Autodesk Fusion 360 part; units mm, degrees
note: some values were not read from the file. Set by a fixed rule: which sketch regions a step uses.
(part 2 of 3)
  line L947 (26.0919, -13.4081) -> (26.0919, -6.5919)
  line L948 (-3.9115, -47.833) -> (-4.0885, -47.833)
  line L949 (-3.9115, -40.0885) -> (-3.9115, -47.833)
  line L950 (-2, -40.0885) -> (-3.9115, -40.0885)
  line L951 (-2, -39.9115) -> (-2, -40.0885)
  line L952 (-3.9115, -39.9115) -> (-2, -39.9115)
  line L953 (-3.9115, -40.0885) -> (-3.9115, -39.9115)
  line L954 (-4.0885, -40.0885) -> (-3.9115, -40.0885)
  line L955 (-4.0885, -39.9115) -> (-4.0885, -40.0885)
  line L956 (-10.9115, -39.9115) -> (-4.0885, -39.9115)
  line L957 (-10.9115, -40.0885) -> (-10.9115, -39.9115)
  line L958 (-11.0885, -40.0885) -> (-10.9115, -40.0885)
  line L959 (-11.0885, -39.9115) -> (-11.0885, -40.0885)
  line L960 (-17.9115, -39.9115) -> (-11.0885, -39.9115)
  line L961 (-17.9115, -40.0885) -> (-17.9115, -39.9115)
  line L962 (-18.0885, -40.0885) -> (-17.9115, -40.0885)
  line L963 (-18.0885, -39.9115) -> (-18.0885, -40.0885)
  line L964 (-17.9115, -39.9115) -> (-18.0885, -39.9115)
  line L965 (-11.0885, -39.9115) -> (-17.9115, -39.9115)
  line L966 (-10.9115, -39.9115) -> (-11.0885, -39.9115)
  line L967 (-4.0885, -39.9115) -> (-10.9115, -39.9115)
  line L968 (-3.9115, -39.9115) -> (-4.0885, -39.9115)
  line L969 (-2, -39.9115) -> (-3.9115, -39.9115)
  line L970 (-3.9115, -39.9115) -> (-2, -39.9115)
  line L971 (-3.9115, -28.0885) -> (-3.9115, -39.9115)
  line L972 (-4.0885, -28.0885) -> (-3.9115, -28.0885)
  line L973 (-4.0885, -39.9115) -> (-4.0885, -28.0885)
  line L974 (-10.9115, -39.9115) -> (-4.0885, -39.9115)
  line L975 (-10.9115, -28.0885) -> (-10.9115, -39.9115)
  line L976 (-11.0885, -28.0885) -> (-10.9115, -28.0885)
  line L977 (-11.0885, -39.9115) -> (-11.0885, -28.0885)
  line L978 (-17.9115, -39.9115) -> (-11.0885, -39.9115)
  line L979 (-17.9115, -28.0885) -> (-17.9115, -39.9115)
  line L980 (-18.0885, -28.0885) -> (-17.9115, -28.0885)
  line L981 (-18.0885, -39.9115) -> (-18.0885, -28.0885)
  line L982 (-24.9115, -39.9115) -> (-18.0885, -39.9115)
  line L983 (-24.9115, -28.0885) -> (-24.9115, -39.9115)
  line L984 (-18.0885, -28.0885) -> (-24.9115, -28.0885)
  line L985 (-17.9115, -28.0885) -> (-18.0885, -28.0885)
  line L986 (-11.0885, -28.0885) -> (-17.9115, -28.0885)
  line L987 (-10.9115, -28.0885) -> (-11.0885, -28.0885)
  line L988 (-4.0885, -28.0885) -> (-10.9115, -28.0885)
  line L989 (-3.9115, -28.0885) -> (-4.0885, -28.0885)
  line L990 (-2, -28.0885) -> (-3.9115, -28.0885)
  line L991 (-2, -27.9115) -> (-2, -28.0885)
  line L992 (-3.9115, -27.9115) -> (-2, -27.9115)
  line L993 (-3.9115, -28.0885) -> (-3.9115, -27.9115)
  line L994 (-4.0885, -28.0885) -> (-3.9115, -28.0885)
  line L995 (-4.0885, -27.9115) -> (-4.0885, -28.0885)
  line L996 (-10.9115, -27.9115) -> (-4.0885, -27.9115)
  line L997 (-10.9115, -28.0885) -> (-10.9115, -27.9115)
  line L998 (-11.0885, -28.0885) -> (-10.9115, -28.0885)
  line L999 (-11.0885, -27.9115) -> (-11.0885, -28.0885)
  line L1000 (-17.9115, -27.9115) -> (-11.0885, -27.9115)
  line L1001 (-17.9115, -28.0885) -> (-17.9115, -27.9115)
  line L1002 (-18.0885, -28.0885) -> (-17.9115, -28.0885)
  line L1003 (-18.0885, -27.9115) -> (-18.0885, -28.0885)
  line L1004 (-24.9115, -27.9115) -> (-18.0885, -27.9115)
  line L1005 (-24.9115, -28.0885) -> (-24.9115, -27.9115)
  line L1006 (-25.0885, -28.0885) -> (-24.9115, -28.0885)
  line L1007 (-25.0885, -27.9115) -> (-25.0885, -28.0885)
  line L1008 (-31.9115, -27.9115) -> (-25.0885, -27.9115)
  line L1009 (-31.9115, -28.0885) -> (-31.9115, -27.9115)
  line L1010 (-32.0885, -28.0885) -> (-31.9115, -28.0885)
  line L1011 (-32.0885, -27.9115) -> (-32.0885, -28.0885)
  line L1012 (-38.9115, -27.9115) -> (-32.0885, -27.9115)
  line L1013 (-38.9115, -27.9821) -> (-38.9115, -27.9115)
  line L1014 (-38.9872, -27.9821) -> (-38.9115, -27.9821)
  line L1015 (-38.9872, -27.9115) -> (-38.9872, -27.9821)
  line L1016 (-38.9115, -27.9115) -> (-38.9872, -27.9115)
  line L1017 (-32.0885, -27.9115) -> (-38.9115, -27.9115)
  line L1018 (-31.9115, -27.9115) -> (-32.0885, -27.9115)
  line L1019 (-25.0885, -27.9115) -> (-31.9115, -27.9115)
  line L1020 (-24.9115, -27.9115) -> (-25.0885, -27.9115)
  line L1021 (-18.0885, -27.9115) -> (-24.9115, -27.9115)
  line L1022 (-17.9115, -27.9115) -> (-18.0885, -27.9115)
  line L1023 (-11.0885, -27.9115) -> (-17.9115, -27.9115)
  line L1024 (-10.9115, -27.9115) -> (-11.0885, -27.9115)
  line L1025 (-4.0885, -27.9115) -> (-10.9115, -27.9115)
  line L1026 (-3.9115, -27.9115) -> (-4.0885, -27.9115)
  line L1027 (-2, -27.9115) -> (-3.9115, -27.9115)
  line L1028 (-3.9115, -27.9115) -> (-2, -27.9115)
  line L1029 (-3.9115, -16.0885) -> (-3.9115, -27.9115)
  line L1030 (-4.0885, -16.0885) -> (-3.9115, -16.0885)
  line L1031 (-4.0885, -27.9115) -> (-4.0885, -16.0885)
  line L1032 (-10.9115, -27.9115) -> (-4.0885, -27.9115)
  line L1033 (-10.9115, -16.0885) -> (-10.9115, -27.9115)
  line L1034 (-11.0885, -16.0885) -> (-10.9115, -16.0885)
  line L1035 (-11.0885, -27.9115) -> (-11.0885, -16.0885)
  line L1036 (-17.9115, -27.9115) -> (-11.0885, -27.9115)
  line L1037 (-17.9115, -16.0885) -> (-17.9115, -27.9115)
  line L1038 (-18.0885, -16.0885) -> (-17.9115, -16.0885)
  line L1039 (-18.0885, -27.9115) -> (-18.0885, -16.0885)
  line L1040 (-24.9115, -27.9115) -> (-18.0885, -27.9115)
  line L1041 (-24.9115, -16.0885) -> (-24.9115, -27.9115)
  line L1042 (-25.0885, -16.0885) -> (-24.9115, -16.0885)
  line L1043 (-25.0885, -27.9115) -> (-25.0885, -16.0885)
  line L1044 (-31.9115, -27.9115) -> (-25.0885, -27.9115)
  line L1045 (-31.9115, -16.0885) -> (-31.9115, -27.9115)
  line L1046 (-32.0885, -16.0885) -> (-31.9115, -16.0885)
  line L1047 (-32.0885, -27.9115) -> (-32.0885, -16.0885)
  line L1048 (-38.9115, -27.9115) -> (-32.0885, -27.9115)
  line L1049 (-38.9115, -16.0885) -> (-38.9115, -27.9115)
  line L1050 (-32.0885, -16.0885) -> (-38.9115, -16.0885)
  line L1051 (-31.9115, -16.0885) -> (-32.0885, -16.0885)
  line L1052 (-25.0885, -16.0885) -> (-31.9115, -16.0885)
  line L1053 (-24.9115, -16.0885) -> (-25.0885, -16.0885)
  line L1054 (-18.0885, -16.0885) -> (-24.9115, -16.0885)
  line L1055 (-17.9115, -16.0885) -> (-18.0885, -16.0885)
  line L1056 (-11.0885, -16.0885) -> (-17.9115, -16.0885)
  line L1057 (-10.9115, -16.0885) -> (-11.0885, -16.0885)
  line L1058 (-4.0885, -16.0885) -> (-10.9115, -16.0885)
  line L1059 (-3.9115, -16.0885) -> (-4.0885, -16.0885)
  line L1060 (-2, -16.0885) -> (-3.9115, -16.0885)
  line L1061 (-2, -15.9115) -> (-2, -16.0885)
  line L1062 (-3.9115, -15.9115) -> (-2, -15.9115)
  line L1063 (-3.9115, -16.0885) -> (-3.9115, -15.9115)
  line L1064 (-4.0885, -16.0885) -> (-3.9115, -16.0885)
  line L1065 (-4.0885, -15.9115) -> (-4.0885, -16.0885)
  line L1066 (-10.9115, -15.9115) -> (-4.0885, -15.9115)
  line L1067 (-10.9115, -16.0885) -> (-10.9115, -15.9115)
  line L1068 (-11.0885, -16.0885) -> (-10.9115, -16.0885)
  line L1069 (-11.0885, -15.9115) -> (-11.0885, -16.0885)
  line L1070 (-17.9115, -15.9115) -> (-11.0885, -15.9115)
  line L1071 (-17.9115, -16.0885) -> (-17.9115, -15.9115)
  line L1072 (-18.0885, -16.0885) -> (-17.9115, -16.0885)
  line L1073 (-18.0885, -15.9115) -> (-18.0885, -16.0885)
  line L1074 (-24.9115, -15.9115) -> (-18.0885, -15.9115)
  line L1075 (-24.9115, -16.0885) -> (-24.9115, -15.9115)
  line L1076 (-25.0885, -16.0885) -> (-24.9115, -16.0885)
  line L1077 (-25.0885, -15.9115) -> (-25.0885, -16.0885)
  line L1078 (-31.9115, -15.9115) -> (-25.0885, -15.9115)
  line L1079 (-31.9115, -16.0885) -> (-31.9115, -15.9115)
  line L1080 (-32.0885, -16.0885) -> (-31.9115, -16.0885)
  line L1081 (-32.0885, -15.9115) -> (-32.0885, -16.0885)
  line L1082 (-31.9115, -15.9115) -> (-32.0885, -15.9115)
  line L1083 (-25.0885, -15.9115) -> (-31.9115, -15.9115)
  line L1084 (-24.9115, -15.9115) -> (-25.0885, -15.9115)
  line L1085 (-18.0885, -15.9115) -> (-24.9115, -15.9115)
  line L1086 (-17.9115, -15.9115) -> (-18.0885, -15.9115)
  line L1087 (-11.0885, -15.9115) -> (-17.9115, -15.9115)
  line L1088 (3.9115, -47.833) -> (3.9115, -40.0885)
  line L1089 (3.9115, -40.0885) -> (2, -40.0885)
  line L1090 (2, -40.0885) -> (2, -39.9115)
  line L1091 (2, -39.9115) -> (3.9115, -39.9115)
  line L1092 (3.9115, -39.9115) -> (3.9115, -40.0885)
  line L1093 (3.9115, -40.0885) -> (4.0885, -40.0885)
  line L1094 (4.0885, -40.0885) -> (4.0885, -39.9115)
  line L1095 (4.0885, -39.9115) -> (10.9115, -39.9115)
  line L1096 (10.9115, -39.9115) -> (10.9115, -40.0885)
  line L1097 (10.9115, -40.0885) -> (11.0885, -40.0885)
  line L1098 (11.0885, -40.0885) -> (11.0885, -39.9115)
  line L1099 (11.0885, -39.9115) -> (17.9115, -39.9115)
  line L1100 (17.9115, -39.9115) -> (17.9115, -40.0885)
  line L1101 (17.9115, -40.0885) -> (18.0885, -40.0885)
  line L1102 (18.0885, -40.0885) -> (18.0885, -39.9115)
  line L1103 (18.0885, -39.9115) -> (17.9115, -39.9115)
  line L1104 (17.9115, -39.9115) -> (11.0885, -39.9115)
  line L1105 (11.0885, -39.9115) -> (10.9115, -39.9115)
  line L1106 (10.9115, -39.9115) -> (4.0885, -39.9115)
  line L1107 (4.0885, -39.9115) -> (3.9115, -39.9115)
  line L1108 (3.9115, -39.9115) -> (2, -39.9115)
  line L1109 (2, -39.9115) -> (3.9115, -39.9115)
  line L1110 (3.9115, -39.9115) -> (3.9115, -28.0885)
  line L1111 (3.9115, -28.0885) -> (4.0885, -28.0885)
  line L1112 (4.0885, -28.0885) -> (4.0885, -39.9115)
  line L1113 (4.0885, -39.9115) -> (10.9115, -39.9115)
  line L1114 (10.9115, -39.9115) -> (10.9115, -28.0885)
  line L1115 (10.9115, -28.0885) -> (11.0885, -28.0885)
  line L1116 (11.0885, -28.0885) -> (11.0885, -39.9115)
  line L1117 (11.0885, -39.9115) -> (17.9115, -39.9115)
  line L1118 (17.9115, -39.9115) -> (17.9115, -28.0885)
  line L1119 (17.9115, -28.0885) -> (18.0885, -28.0885)
  line L1120 (18.0885, -28.0885) -> (18.0885, -39.9115)
  line L1121 (18.0885, -39.9115) -> (24.9115, -39.9115)
  line L1122 (24.9115, -39.9115) -> (24.9115, -28.0885)
  line L1123 (24.9115, -28.0885) -> (18.0885, -28.0885)
  line L1124 (18.0885, -28.0885) -> (17.9115, -28.0885)
  line L1125 (17.9115, -28.0885) -> (11.0885, -28.0885)
  line L1126 (11.0885, -28.0885) -> (10.9115, -28.0885)
  line L1127 (10.9115, -28.0885) -> (4.0885, -28.0885)
  line L1128 (4.0885, -28.0885) -> (3.9115, -28.0885)
  line L1129 (3.9115, -28.0885) -> (2, -28.0885)
  line L1130 (2, -28.0885) -> (2, -27.9115)
  line L1131 (2, -27.9115) -> (3.9115, -27.9115)
  line L1132 (3.9115, -27.9115) -> (3.9115, -28.0885)
  line L1133 (3.9115, -28.0885) -> (4.0885, -28.0885)
  line L1134 (4.0885, -28.0885) -> (4.0885, -27.9115)
  line L1135 (4.0885, -27.9115) -> (10.9115, -27.9115)
  line L1136 (10.9115, -27.9115) -> (10.9115, -28.0885)
  line L1137 (10.9115, -28.0885) -> (11.0885, -28.0885)
  line L1138 (11.0885, -28.0885) -> (11.0885, -27.9115)
  line L1139 (11.0885, -27.9115) -> (17.9115, -27.9115)
  line L1140 (17.9115, -27.9115) -> (17.9115, -28.0885)
  line L1141 (17.9115, -28.0885) -> (18.0885, -28.0885)
  line L1142 (18.0885, -28.0885) -> (18.0885, -27.9115)
  line L1143 (18.0885, -27.9115) -> (24.9115, -27.9115)
  line L1144 (24.9115, -27.9115) -> (24.9115, -28.0885)
  line L1145 (24.9115, -28.0885) -> (25.0885, -28.0885)
  line L1146 (25.0885, -28.0885) -> (25.0885, -27.9115)
  line L1147 (25.0885, -27.9115) -> (31.9115, -27.9115)
  line L1148 (31.9115, -27.9115) -> (31.9115, -28.0885)
  line L1149 (31.9115, -28.0885) -> (32.0885, -28.0885)
  line L1150 (32.0885, -28.0885) -> (32.0885, -27.9115)
  line L1151 (32.0885, -27.9115) -> (38.9115, -27.9115)
  line L1152 (38.9115, -27.9115) -> (38.9115, -27.9821)
  line L1153 (38.9115, -27.9821) -> (38.9872, -27.9821)
  line L1154 (38.9872, -27.9821) -> (38.9872, -27.9115)
  line L1155 (38.9872, -27.9115) -> (38.9115, -27.9115)
  line L1156 (38.9115, -27.9115) -> (32.0885, -27.9115)
  line L1157 (32.0885, -27.9115) -> (31.9115, -27.9115)
  line L1158 (31.9115, -27.9115) -> (25.0885, -27.9115)
  line L1159 (25.0885, -27.9115) -> (24.9115, -27.9115)
  line L1160 (24.9115, -27.9115) -> (18.0885, -27.9115)
  line L1161 (18.0885, -27.9115) -> (17.9115, -27.9115)
  line L1162 (17.9115, -27.9115) -> (11.0885, -27.9115)
  line L1163 (11.0885, -27.9115) -> (10.9115, -27.9115)
  line L1164 (10.9115, -27.9115) -> (4.0885, -27.9115)
  line L1165 (4.0885, -27.9115) -> (3.9115, -27.9115)
  line L1166 (3.9115, -27.9115) -> (2, -27.9115)
  line L1167 (2, -27.9115) -> (3.9115, -27.9115)
  line L1168 (3.9115, -27.9115) -> (3.9115, -16.0885)
  line L1169 (3.9115, -16.0885) -> (4.0885, -16.0885)
  line L1170 (4.0885, -16.0885) -> (4.0885, -27.9115)
  line L1171 (4.0885, -27.9115) -> (10.9115, -27.9115)
  line L1172 (10.9115, -27.9115) -> (10.9115, -16.0885)
  line L1173 (10.9115, -16.0885) -> (11.0885, -16.0885)
  line L1174 (11.0885, -16.0885) -> (11.0885, -27.9115)
  line L1175 (11.0885, -27.9115) -> (17.9115, -27.9115)
  line L1176 (17.9115, -27.9115) -> (17.9115, -16.0885)
  line L1177 (17.9115, -16.0885) -> (18.0885, -16.0885)
  line L1178 (18.0885, -16.0885) -> (18.0885, -27.9115)
  line L1179 (18.0885, -27.9115) -> (24.9115, -27.9115)
  line L1180 (24.9115, -27.9115) -> (24.9115, -16.0885)
  line L1181 (24.9115, -16.0885) -> (25.0885, -16.0885)
  line L1182 (25.0885, -16.0885) -> (25.0885, -27.9115)
  line L1183 (25.0885, -27.9115) -> (31.9115, -27.9115)
  line L1184 (31.9115, -27.9115) -> (31.9115, -16.0885)
  line L1185 (31.9115, -16.0885) -> (32.0885, -16.0885)
  line L1186 (32.0885, -16.0885) -> (32.0885, -27.9115)
  line L1187 (32.0885, -27.9115) -> (38.9115, -27.9115)
  line L1188 (38.9115, -27.9115) -> (38.9115, -16.0885)
  line L1189 (38.9115, -16.0885) -> (32.0885, -16.0885)
  line L1190 (32.0885, -16.0885) -> (31.9115, -16.0885)
  line L1191 (31.9115, -16.0885) -> (25.0885, -16.0885)
  line L1192 (25.0885, -16.0885) -> (24.9115, -16.0885)
  line L1193 (24.9115, -16.0885) -> (18.0885, -16.0885)
  line L1194 (18.0885, -16.0885) -> (17.9115, -16.0885)
  line L1195 (17.9115, -16.0885) -> (11.0885, -16.0885)
  line L1196 (11.0885, -16.0885) -> (10.9115, -16.0885)
  line L1197 (10.9115, -16.0885) -> (4.0885, -16.0885)
  line L1198 (4.0885, -16.0885) -> (3.9115, -16.0885)
  line L1199 (3.9115, -16.0885) -> (2, -16.0885)
  line L1200 (2, -16.0885) -> (2, -15.9115)
  line L1201 (2, -15.9115) -> (3.9115, -15.9115)
  line L1202 (3.9115, -15.9115) -> (3.9115, -16.0885)
  line L1203 (3.9115, -16.0885) -> (4.0885, -16.0885)
  line L1204 (4.0885, -16.0885) -> (4.0885, -15.9115)
  line L1205 (4.0885, -15.9115) -> (10.9115, -15.9115)
  line L1206 (10.9115, -15.9115) -> (10.9115, -16.0885)
  line L1207 (10.9115, -16.0885) -> (11.0885, -16.0885)
  line L1208 (11.0885, -16.0885) -> (11.0885, -15.9115)
  line L1209 (11.0885, -15.9115) -> (17.9115, -15.9115)
  line L1210 (17.9115, -15.9115) -> (17.9115, -16.0885)
  line L1211 (17.9115, -16.0885) -> (18.0885, -16.0885)
  line L1212 (18.0885, -16.0885) -> (18.0885, -15.9115)
  line L1213 (18.0885, -15.9115) -> (24.9115, -15.9115)
  line L1214 (24.9115, -15.9115) -> (24.9115, -16.0885)
  line L1215 (24.9115, -16.0885) -> (25.0885, -16.0885)
  line L1216 (25.0885, -16.0885) -> (25.0885, -15.9115)
  line L1217 (-24.9115, -3.9115) -> (-25.0885, -3.9115)
  line L1218 (-32.0885, -2) -> (-31.9115, -2)
  line L1219 (-17.9115, -3.9115) -> (-11.0885, -3.9115)
  line L1220 (-4.0885, -4.0885) -> (-3.9115, -4.0885)
  line L1221 (-2, -4.0885) -> (-3.9115, -4.0885)
  line L1222 (-3.9115, -3.9115) -> (-4.0885, -3.9115)
  line L1223 (-11.0885, -4.0885) -> (-17.9115, -4.0885)
  line L1224 (-25.0885, -4.0885) -> (-31.9115, -4.0885)
  line L1225 (-18.0885, -40.0885) -> (-24.9115, -40.0885)
  line L1226 (-18.0885, -3.9115) -> (-18.0885, -4.0885)
  line L1227 (-38.9872, -28.0885) -> (-38.9872, -27.9821)
  line L1228 (-31.9115, -3.9115) -> (-32.0885, -3.9115)
  line L1229 (-38.9115, -3.9115) -> (-39.0885, -3.9115)
  line L1230 (-45.9115, -3.9115) -> (-39.0885, -3.9115)
  line L1231 (-38.9115, -15.9115) -> (-39.0885, -15.9115)
  line L1232 (-45.9115, -4.0885) -> (-45.9115, -3.9115)
  line L1233 (-3.9115, -3.9115) -> (-2, -3.9115)
  line L1234 (-18.0885, -3.9115) -> (-24.9115, -3.9115)
  line L1235 (-38.9115, -15.9115) -> (-32.0885, -15.9115)
  line L1236 (-31.9115, -35.7771) -> (-32.0885, -35.7771)
  line L1237 (-32.0885, -28.0885) -> (-38.9872, -28.0885)
  line L1238 (-31.9115, -28.0885) -> (-31.9115, -35.7771)
  line L1239 (-18.0885, -15.9115) -> (-18.0885, -4.0885)
  line L1240 (-3.9115, -2) -> (-3.9115, -3.9115)
  line L1241 (-11.0885, -3.9115) -> (-11.0885, -2)
  line L1242 (-24.9115, -4.0885) -> (-25.0885, -4.0885)
  line L1243 (-4.0885, -4.0885) -> (-10.9115, -4.0885)
  line L1244 (-18.0885, -4.0885) -> (-17.9115, -4.0885)
  line L1245 (-11.0885, -4.0885) -> (-10.9115, -4.0885)
  line L1246 (-31.9115, -3.9115) -> (-25.0885, -3.9115)
  line L1247 (-10.9115, -3.9115) -> (-11.0885, -3.9115)
  line L1248 (-25.0885, -3.9115) -> (-25.0885, -2)
  line L1249 (-2, -3.9115) -> (-2, -4.0885)
  line L1250 (-17.9115, -40.0885) -> (-17.9115, -44.4972)
  line L1251 (-18.0885, -4.0885) -> (-17.9115, -4.0885)
  line L1252 (-47.833, -4.0885) -> (-47.833, -3.9115)
  line L1253 (-3.9115, -4.0885) -> (-4.0885, -4.0885)
  line L1254 (-38.9115, -3.9115) -> (-32.0885, -3.9115)
  line L1255 (-31.9115, -4.0885) -> (-31.9115, -3.9115)
  line L1256 (-39.0885, -16.0885) -> (-45.2548, -16.0885)
  line L1257 (-3.9115, -3.9115) -> (-2, -3.9115)
  line L1258 (-3.9115, -15.9115) -> (-2, -15.9115)
  line L1259 (-32.0885, -3.9115) -> (-38.9115, -3.9115)
  line L1260 (-4.0885, -3.9115) -> (-10.9115, -3.9115)
  line L1261 (-31.9115, -3.9115) -> (-25.0885, -3.9115)
  line L1262 (-32.0885, -3.9115) -> (-32.0885, -2)
  line L1263 (-3.9115, -4.0885) -> (-3.9115, -3.9115)
  line L1264 (-24.9115, -2) -> (-24.9115, -3.9115)
  line L1265 (-31.9115, -15.9115) -> (-25.0885, -15.9115)
  line L1266 (-17.9115, -2) -> (-17.9115, -3.9115)
  line L1267 (-39.0885, -27.9821) -> (-39.0885, -16.0885)
  line L1268 (-26.533, -40.0885) -> (-26.533, -39.9115)
  line L1269 (-46.0885, -3.9115) -> (-46.0885, -4.0885)
  line L1270 (-47.833, -3.9115) -> (-46.0885, -3.9115)
  line L1271 (-17.9115, -3.9115) -> (-18.0885, -3.9115)
  line L1272 (-45.9115, -4.0885) -> (-45.9115, -13.7113)
  line L1273 (-10.9115, -3.9115) -> (-4.0885, -3.9115)
  line L1274 (-25.0885, -40.9756) -> (-25.0885, -40.0885)
  line L1275 (-39.0885, -3.9115) -> (-39.0885, -4.0885)
  line L1276 (-17.9115, -4.0885) -> (-18.0885, -4.0885)
  line L1277 (-11.0885, -15.9115) -> (-11.0885, -4.0885)
  line L1278 (-38.9115, -16.0885) -> (-38.9115, -15.9115)
  line L1279 (-18.0885, -2) -> (-17.9115, -2)
  line L1280 (-4.0885, -4.0885) -> (-3.9115, -4.0885)
  line L1281 (-38.9115, -4.0885) -> (-38.9115, -3.9115)
  line L1282 (-32.0885, -4.0885) -> (-38.9115, -4.0885)
  line L1283 (-46.0885, -4.0885) -> (-45.9115, -4.0885)
  line L1284 (-25.0885, -3.9115) -> (-31.9115, -3.9115)
  line L1285 (-24.9115, -3.9115) -> (-18.0885, -3.9115)
  line L1286 (-24.9115, -39.9115) -> (-25.0885, -39.9115)
  line L1287 (-26.533, -39.9115) -> (-25.0885, -39.9115)
  line L1288 (-39.0885, -15.9115) -> (-39.0885, -16.0885)
  line L1289 (-24.9115, -4.0885) -> (-24.9115, -3.9115)
  line L1290 (-25.0885, -39.9115) -> (-25.0885, -40.0885)
  line L1291 (-10.9115, -4.0885) -> (-10.9115, -3.9115)
  line L1292 (-31.9115, -4.0885) -> (-32.0885, -4.0885)
  line L1293 (-25.0885, -40.0885) -> (-24.9115, -40.0885)
  line L1294 (-25.0885, -4.0885) -> (-24.9115, -4.0885)
  line L1295 (-38.9872, -27.9821) -> (-39.0885, -27.9821)
  line L1296 (-45.2548, -16.0885) -> (-45.2548, -15.9115)
  line L1297 (-11.0885, -3.9115) -> (-17.9115, -3.9115)
  line L1298 (-32.0885, -15.9115) -> (-32.0885, -4.0885)
  line L1299 (-25.0885, -40.0885) -> (-26.533, -40.0885)
  line L1300 (-45.9115, -2) -> (-45.9115, -3.9115)
  line L1301 (-45.2548, -15.9115) -> (-39.0885, -15.9115)
  line L1302 (-11.0885, -2) -> (-10.9115, -2)
  line L1303 (-46.0885, -13.7113) -> (-46.0885, -4.0885)
  line L1304 (-38.9115, -3.9115) -> (-32.0885, -3.9115)
  line L1305 (-24.9115, -4.0885) -> (-24.9115, -15.9115)
  line L1306 (-25.0885, -4.0885) -> (-24.9115, -4.0885)
  line L1307 (-17.9115, -3.9115) -> (-11.0885, -3.9115)
  line L1308 (-18.0885, -44.4972) -> (-18.0885, -40.0885)
  line L1309 (-10.9115, -4.0885) -> (-10.9115, -15.9115)
  line L1310 (-24.9115, -40.0885) -> (-24.9115, -39.9115)
  line L1311 (-32.0885, -35.7771) -> (-32.0885, -28.0885)
  line L1312 (-18.0885, -4.0885) -> (-24.9115, -4.0885)
  line L1313 (-25.0885, -28.0885) -> (-31.9115, -28.0885)
  line L1314 (-17.9115, -4.0885) -> (-17.9115, -15.9115)
  line L1315 (-17.9115, -44.4972) -> (-18.0885, -44.4972)
  line L1316 (-31.9115, -2) -> (-31.9115, -3.9115)
  line L1317 (-46.0885, -4.0885) -> (-47.833, -4.0885)
  line L1318 (-24.9115, -3.9115) -> (-18.0885, -3.9115)
  line L1319 (-39.0885, -4.0885) -> (-38.9115, -4.0885)
  line L1320 (-25.0885, -2) -> (-24.9115, -2)
  line L1321 (-18.0885, -3.9115) -> (-18.0885, -2)
  line L1322 (-45.9115, -13.7113) -> (-46.0885, -13.7113)
  line L1323 (-2, -3.9115) -> (-3.9115, -3.9115)
  line L1324 (-24.9115, -15.9115) -> (-18.0885, -15.9115)
  line L1325 (-32.0885, -4.0885) -> (-31.9115, -4.0885)
  line L1326 (-38.9115, -4.0885) -> (-38.9115, -15.9115)
  line L1327 (-11.0885, -4.0885) -> (-10.9115, -4.0885)
  line L1328 (-25.0885, -39.9115) -> (-25.0885, -28.0885)
  line L1329 (-24.9115, -40.0885) -> (-24.9115, -40.9756)
  line L1330 (-45.9115, -3.9115) -> (-46.0885, -3.9115)
  line L1331 (-39.0885, -3.9115) -> (-39.0885, -2)
  line L1332 (-10.9115, -15.9115) -> (-4.0885, -15.9115)
  line L1333 (-4.0885, -2) -> (-3.9115, -2)
  line L1334 (-39.0885, -4.0885) -> (-45.9115, -4.0885)
  line L1335 (-46.0885, -2) -> (-45.9115, -2)
  line L1336 (-17.9115, -4.0885) -> (-17.9115, -3.9115)
  line L1337 (-46.0885, -3.9115) -> (-46.0885, -2)
  line L1338 (-38.9115, -2) -> (-38.9115, -3.9115)
  line L1339 (-25.0885, -15.9115) -> (-25.0885, -4.0885)
  line L1340 (-10.9115, -2) -> (-10.9115, -3.9115)
  line L1341 (-32.0885, -3.9115) -> (-32.0885, -4.0885)
  line L1342 (-31.9115, -4.0885) -> (-31.9115, -15.9115)
  line L1343 (-17.9115, -15.9115) -> (-11.0885, -15.9115)
  line L1344 (-39.0885, -2) -> (-38.9115, -2)
  line L1345 (-32.0885, -4.0885) -> (-31.9115, -4.0885)
  line L1346 (-10.9115, -4.0885) -> (-11.0885, -4.0885)
  line L1347 (-24.9115, -40.9756) -> (-25.0885, -40.9756)
  line L1348 (-4.0885, -15.9115) -> (-4.0885, -4.0885)
  line L1349 (-10.9115, -3.9115) -> (-4.0885, -3.9115)
  line L1350 (-11.0885, -3.9115) -> (-11.0885, -4.0885)
  line L1351 (-4.0885, -3.9115) -> (-4.0885, -2)
  line L1352 (-25.0885, -3.9115) -> (-25.0885, -4.0885)
  line L1353 (-39.0885, -15.9115) -> (-39.0885, -4.0885)
  line L1354 (-39.0885, -16.0885) -> (-38.9115, -16.0885)
  line L1355 (-3.9115, -4.0885) -> (-3.9115, -15.9115)
  line L1356 (-4.0885, -3.9115) -> (-4.0885, -4.0885)
  line L1357 (-3.9115, -15.9115) -> (-4.0885, -15.9115)
  line L1358 (-4.0885, -15.9115) -> (-10.9115, -15.9115)
  line L1359 (-2, -15.9115) -> (-3.9115, -15.9115)
  line L1360 (21.1309, 45.3154) -> (23.0874, 44.3505)
  line L1361 (-33.5, -7) -> (-33.5, -13)
  line L1362 (-48.8148, 10.822) -> (-48.2963, 12.941)
  line L1363 (-33.5, -13) -> (-37.5, -13)
  line L1364 (-26.5, 19) -> (-30.5, 19)
  line L1365 (30.5, 19) -> (26.5, 19)
  line L1366 (-5.5, 13) -> (-5.5, 7)
  line L1367 (-30.5, 19) -> (-30.5, 25)
  line L1368 (-9.5, 13) -> (-5.5, 13)
  line L1369 (-30.5, 25) -> (-26.5, 25)
  line L1370 (30.5, 25) -> (30.5, 19)
  line L1371 (-9.5, 7) -> (-9.5, 13)
  line L1372 (37.5, 7) -> (33.5, 7)
  line L1373 (-37.5, -7) -> (-33.5, -7)
  line L1374 (33.5, 13) -> (37.5, 13)
  line L1375 (-5.5, -19) -> (-5.5, -25)
  line L1376 (37.5, 13) -> (37.5, 7)
  line L1377 (-37.5, -13) -> (-37.5, -7)
  line L1378 (-5.5, 7) -> (-9.5, 7)
  line L1379 (-5.5, -25) -> (-9.5, -25)
  line L1380 (-48.2963, 12.941) -> (-47.6858, 15.0353)
  line L1381 (26.5, 25) -> (30.5, 25)
  line L1382 (26.5, 19) -> (26.5, 25)
  line L1383 (-26.5, 25) -> (-26.5, 19)
  line L1384 (-9.5, -19) -> (-5.5, -19)
  line L1385 (-9.5, -25) -> (-9.5, -19)
  line L1386 (23.5, -37) -> (19.5, -37)
  line L1387 (-48.2963, -12.941) -> (-48.8148, -10.822)
  line L1388 (-42.1696, -26.865) -> (-43.3013, -25)
  line L1389 (-46.194, -19.1342) -> (-46.9846, -17.101)
  line L1390 (-46.9846, -17.101) -> (-47.6858, -15.0353)
  line L1391 (-45.3154, -21.1309) -> (-46.194, -19.1342)
  line L1392 (-44.3505, -23.0874) -> (-45.3154, -21.1309)
  line L1393 (-43.3013, -25) -> (-44.3505, -23.0874)
  line L1394 (-47.6858, -15.0353) -> (-48.2963, -12.941)
  line L1395 (-39.6677, -30.4381) -> (-40.9576, -28.6788)
  line L1396 (-40.9576, -28.6788) -> (-42.1696, -26.865)
  line L1397 (-38.3022, -32.1394) -> (-39.6677, -30.4381)
  line L1398 (43.3013, -25) -> (42.1696, -26.865)
  line L1399 (-49.5722, -6.5263) -> (-49.8097, -4.3578)
  line L1400 (40.9576, -28.6788) -> (39.6677, -30.4381)
  line L1401 (39.6677, -30.4381) -> (38.3022, -32.1394)
  line L1402 (32.1394, -38.3022) -> (30.4381, -39.6677)
  line L1403 (49.8097, -4.3578) -> (49.5722, -6.5263)
  line L1404 (48.8148, -10.822) -> (48.2963, -12.941)
  line L1405 (38.3022, -32.1394) -> (36.8639, -33.7795)
  line L1406 (0, 0) -> (0, -50)
  line L1407 (-48.8148, -10.822) -> (-49.2404, -8.6824)
  line L1408 (33.7795, -36.8639) -> (32.1394, -38.3022)
  line L1409 (36.8639, -33.7795) -> (35.3553, -35.3553)
  line L1410 (35.3553, -35.3553) -> (33.7795, -36.8639)
  line L1411 (49.9524, -2.181) -> (49.8097, -4.3578)
  line L1412 (0, -50) -> (0, 0)
  line L1413 (46.9846, -17.101) -> (46.194, -19.1342)
  line L1414 (42.1696, -26.865) -> (40.9576, -28.6788)
  line L1415 (46.194, -19.1342) -> (45.3154, -21.1309)
  line L1416 (-49.9524, -2.181) -> (-50, 0)
  line L1417 (45.3154, -21.1309) -> (44.3505, -23.0874)
  line L1418 (44.3505, -23.0874) -> (43.3013, -25)
  line L1419 (-49.8097, -4.3578) -> (-49.9524, -2.181)
  line L1420 (0, 0) -> (50, 0)
  line L1421 (50, 0) -> (49.9524, -2.181)
  line L1422 (48.2963, -12.941) -> (47.6858, -15.0353)
  line L1423 (49.2404, -8.6824) -> (48.8148, -10.822)
  line L1424 (-49.2404, -8.6824) -> (-49.5722, -6.5263)
  line L1425 (47.6858, -15.0353) -> (46.9846, -17.101)
  line L1426 (-50, 0) -> (0, 0)
  line L1427 (49.5722, -6.5263) -> (49.2404, -8.6824)
  line L1428 (23.0874, -44.3505) -> (21.1309, -45.3154)
  line L1429 (26.865, -42.1696) -> (25, -43.3013)
  line L1430 (30.4381, -39.6677) -> (28.6788, -40.9576)
  line L1431 (28.6788, -40.9576) -> (26.865, -42.1696)
  line L1432 (25, -43.3013) -> (23.0874, -44.3505)
  line L1433 (21.1309, -45.3154) -> (19.1342, -46.194)
  line L1434 (17.101, -46.9846) -> (15.0353, -47.6858)
  line L1435 (15.0353, -47.6858) -> (12.941, -48.2963)
  line L1436 (10.822, -48.8148) -> (8.6824, -49.2404)
  line L1437 (12.941, -48.2963) -> (10.822, -48.8148)
  line L1438 (8.6824, -49.2404) -> (6.5263, -49.5722)
  line L1439 (19.1342, -46.194) -> (17.101, -46.9846)
  line L1440 (36.8639, -33.7795) -> (35.3553, -35.3553)
  line L1441 (5.5, -13) -> (5.5, -7)
  line L1442 (26.865, -42.1696) -> (25, -43.3013)
  line L1443 (40.9576, -28.6788) -> (39.6677, -30.4381)
  line L1444 (8.6824, -49.2404) -> (6.5263, -49.5722)
  line L1445 (17.101, -46.9846) -> (15.0353, -47.6858)
  line L1446 (38.3022, -32.1394) -> (36.8639, -33.7795)
  line L1447 (23.0874, -44.3505) -> (21.1309, -45.3154)
  line L1448 (15.0353, -47.6858) -> (12.941, -48.2963)
  line L1449 (30.4381, -39.6677) -> (28.6788, -40.9576)
  line L1450 (43.3013, -25) -> (42.1696, -26.865)
  line L1451 (2.181, -49.9524) -> (0, -50)
  line L1452 (28.6788, -40.9576) -> (26.865, -42.1696)
  line L1453 (19.1342, -46.194) -> (17.101, -46.9846)
  line L1454 (19.5, -31) -> (23.5, -31)
  line L1455 (5.5, -7) -> (9.5, -7)
  line L1456 (35.3553, -35.3553) -> (33.7795, -36.8639)
  line L1457 (19.5, -37) -> (19.5, -31)
  line L1458 (44.3505, -23.0874) -> (43.3013, -25)
  line L1459 (6.5263, -49.5722) -> (4.3578, -49.8097)
  line L1460 (33.7795, -36.8639) -> (32.1394, -38.3022)
  line L1461 (4.3578, -49.8097) -> (2.181, -49.9524)
  line L1462 (9.5, -7) -> (9.5, -13)
  line L1463 (32.1394, -38.3022) -> (30.4381, -39.6677)
  line L1464 (21.1309, -45.3154) -> (19.1342, -46.194)
  line L1465 (45.3154, -21.1309) -> (44.3505, -23.0874)
  line L1466 (9.5, -13) -> (5.5, -13)
  line L1467 (39.6677, -30.4381) -> (38.3022, -32.1394)
  line L1468 (12.941, -48.2963) -> (10.822, -48.8148)
  line L1469 (10.822, -48.8148) -> (8.6824, -49.2404)
  line L1470 (25, -43.3013) -> (23.0874, -44.3505)
  line L1471 (23.5, -31) -> (23.5, -37)
  line L1472 (42.1696, -26.865) -> (40.9576, -28.6788)
  line L1473 (49.2404, -8.6824) -> (48.8148, -10.822)
  line L1474 (46.9846, 17.101) -> (47.6858, 15.0353)
  line L1475 (48.2963, 12.941) -> (48.8148, 10.822)
  line L1476 (35.3553, 35.3553) -> (36.8639, 33.7795)
  line L1477 (42.1696, 26.865) -> (43.3013, 25)
  line L1478 (45.3154, 21.1309) -> (46.194, 19.1342)
  line L1479 (49.8097, -4.3578) -> (49.5722, -6.5263)
  line L1480 (39.6677, 30.4381) -> (40.9576, 28.6788)
  line L1481 (48.8148, 10.822) -> (49.2404, 8.6824)
  line L1482 (49.5722, 6.5263) -> (49.8097, 4.3578)
  line L1483 (49.9524, 2.181) -> (50, 0)
  line L1484 (46.194, -19.1342) -> (45.3154, -21.1309)
  line L1485 (47.6858, -15.0353) -> (46.9846, -17.101)
  line L1486 (49.8097, 4.3578) -> (49.9524, 2.181)
  line L1487 (49.5722, -6.5263) -> (49.2404, -8.6824)
  line L1488 (38.3022, 32.1394) -> (39.6677, 30.4381)
  line L1489 (48.2963, -12.941) -> (47.6858, -15.0353)
  line L1490 (46.9846, -17.101) -> (46.194, -19.1342)
  line L1491 (36.8639, 33.7795) -> (38.3022, 32.1394)
  line L1492 (47.6858, 15.0353) -> (48.2963, 12.941)
  line L1493 (33.7795, 36.8639) -> (35.3553, 35.3553)
  line L1494 (43.3013, 25) -> (44.3505, 23.0874)
  line L1495 (50, 0) -> (49.9524, -2.181)
  line L1496 (48.8148, -10.822) -> (48.2963, -12.941)
  line L1497 (40.9576, 28.6788) -> (42.1696, 26.865)
  line L1498 (46.194, 19.1342) -> (46.9846, 17.101)
  line L1499 (49.9524, -2.181) -> (49.8097, -4.3578)
  line L1500 (44.3505, 23.0874) -> (45.3154, 21.1309)
  line L1501 (49.2404, 8.6824) -> (49.5722, 6.5263)
  line L1502 (32.1394, 38.3022) -> (33.7795, 36.8639)
  line L1503 (48.8148, 10.822) -> (49.2404, 8.6824)
  line L1504 (-4.3578, -49.8097) -> (-6.5263, -49.5722)
  line L1505 (-43.3013, 25) -> (-42.1696, 26.865)
  line L1506 (-17.101, 46.9846) -> (-15.0353, 47.6858)
  line L1507 (-49.9524, 2.181) -> (-49.8097, 4.3578)
  line L1508 (-4.3578, 49.8097) -> (-2.181, 49.9524)
  line L1509 (46.9846, 17.101) -> (47.6858, 15.0353)
  line L1510 (-2.181, 49.9524) -> (0, 50)
  line L1511 (8.6824, 49.2404) -> (10.822, 48.8148)
  line L1512 (-49.2404, 8.6824) -> (-48.8148, 10.822)
  line L1513 (-10.822, 48.8148) -> (-8.6824, 49.2404)
  line L1514 (-44.3505, 23.0874) -> (-43.3013, 25)
  line L1515 (-8.6824, 49.2404) -> (-6.5263, 49.5722)
  line L1516 (47.6858, 15.0353) -> (48.2963, 12.941)
  line L1517 (46.194, 19.1342) -> (46.9846, 17.101)
  line L1518 (-49.8097, -4.3578) -> (-49.9524, -2.181)
  line L1519 (-49.5722, 6.5263) -> (-49.2404, 8.6824)
  line L1520 (43.3013, 25) -> (44.3505, 23.0874)
  line L1521 (-25, 43.3013) -> (-23.0874, 44.3505)
  line L1522 (-46.9846, 17.101) -> (-46.194, 19.1342)
  line L1523 (-50, 0) -> (-49.9524, 2.181)
  line L1524 (33.5, 7) -> (33.5, 13)
  line L1525 (-30.4381, 39.6677) -> (-28.6788, 40.9576)
  line L1526 (-49.8097, 4.3578) -> (-49.5722, 6.5263)
  line L1527 (-6.5263, 49.5722) -> (-4.3578, 49.8097)
  line L1528 (-26.865, 42.1696) -> (-25, 43.3013)
  line L1529 (-42.1696, 26.865) -> (-40.9576, 28.6788)
  line L1530 (-39.6677, 30.4381) -> (-38.3022, 32.1394)
  line L1531 (0, -50) -> (-2.181, -49.9524)
  line L1532 (44.3505, 23.0874) -> (45.3154, 21.1309)
  line L1533 (-33.7795, 36.8639) -> (-32.1394, 38.3022)
  line L1534 (19.1342, 46.194) -> (21.1309, 45.3154)
  line L1535 (-46.9846, -17.101) -> (-47.6858, -15.0353)
  line L1536 (-12.941, 48.2963) -> (-10.822, 48.8148)
  line L1537 (-35.3553, 35.3553) -> (-33.7795, 36.8639)
  line L1538 (-19.1342, 46.194) -> (-17.101, 46.9846)
  line L1539 (17.101, 46.9846) -> (19.1342, 46.194)
  line L1540 (6.5263, 49.5722) -> (8.6824, 49.2404)
  line L1541 (-49.8097, 4.3578) -> (-49.5722, 6.5263)
  line L1542 (40.9576, 28.6788) -> (42.1696, 26.865)
  line L1543 (-38.3022, 32.1394) -> (-36.8639, 33.7795)
  line L1544 (48.2963, 12.941) -> (48.8148, 10.822)
  line L1545 (-23.0874, 44.3505) -> (-21.1309, 45.3154)
  line L1546 (42.1696, 26.865) -> (43.3013, 25)
  line L1547 (-49.5722, 6.5263) -> (-49.2404, 8.6824)
  line L1548 (49.2404, 8.6824) -> (49.5722, 6.5263)
  line L1549 (-48.8148, -10.822) -> (-49.2404, -8.6824)
  line L1550 (15.0353, 47.6858) -> (17.101, 46.9846)
  line L1551 (-21.1309, 45.3154) -> (-19.1342, 46.194)
  line L1552 (-28.6788, 40.9576) -> (-26.865, 42.1696)
  line L1553 (45.3154, 21.1309) -> (46.194, 19.1342)
  line L1554 (49.5722, 6.5263) -> (49.8097, 4.3578)
  line L1555 (-2.181, -49.9524) -> (-4.3578, -49.8097)
  line L1556 (-49.9524, -2.181) -> (-50, 0)
  line L1557 (-40.9576, 28.6788) -> (-39.6677, 30.4381)
  line L1558 (39.6677, 30.4381) -> (40.9576, 28.6788)
  line L1559 (-47.6858, -15.0353) -> (-48.2963, -12.941)
  line L1560 (-48.2963, 12.941) -> (-47.6858, 15.0353)
  line L1561 (-49.2404, 8.6824) -> (-48.8148, 10.822)
  line L1562 (-44.3505, -23.0874) -> (-45.3154, -21.1309)
  line L1563 (-50, 0) -> (-49.9524, 2.181)
  line L1564 (-43.3013, -25) -> (-44.3505, -23.0874)
  line L1565 (-30.4381, -39.6677) -> (-32.1394, -38.3022)
  line L1566 (49.8097, 4.3578) -> (49.9524, 2.181)
  line L1567 (-15.0353, -47.6858) -> (-17.101, -46.9846)
  line L1568 (10.822, 48.8148) -> (12.941, 48.2963)
  line L1569 (-36.8639, -33.7795) -> (-38.3022, -32.1394)
  line L1570 (-49.5722, -6.5263) -> (-49.8097, -4.3578)
  line L1571 (-21.1309, -45.3154) -> (-23.0874, -44.3505)
  line L1572 (50, 0) -> (0, 0)
  line L1573 (-49.9524, 2.181) -> (-49.8097, 4.3578)
  line L1574 (-36.8639, 33.7795) -> (-35.3553, 35.3553)
  line L1575 (0, 0) -> (-50, 0)
  line L1576 (-6.5263, -49.5722) -> (-8.6824, -49.2404)
  line L1577 (-12.941, -48.2963) -> (-15.0353, -47.6858)
  line L1578 (-48.2963, -12.941) -> (-48.8148, -10.822)
  line L1579 (-49.2404, -8.6824) -> (-49.5722, -6.5263)
  line L1580 (28.6788, 40.9576) -> (30.4381, 39.6677)
  line L1581 (-32.1394, -38.3022) -> (-33.7795, -36.8639)
  line L1582 (-38.3022, -32.1394) -> (-39.6677, -30.4381)
  line L1583 (-10.822, -48.8148) -> (-12.941, -48.2963)
  line L1584 (26.865, 42.1696) -> (28.6788, 40.9576)
  line L1585 (-40.9576, -28.6788) -> (-42.1696, -26.865)
  line L1586 (-46.194, -19.1342) -> (-46.9846, -17.101)
  line L1587 (-35.3553, -35.3553) -> (-36.8639, -33.7795)
  line L1588 (-39.6677, -30.4381) -> (-40.9576, -28.6788)
  line L1589 (-42.1696, -26.865) -> (-43.3013, -25)
  line L1590 (-45.3154, -21.1309) -> (-46.194, -19.1342)
  line L1591 (36.8639, 33.7795) -> (38.3022, 32.1394)
  line L1592 (-47.6858, 15.0353) -> (-46.9846, 17.101)
  line L1593 (49.9524, 2.181) -> (50, 0)
  line L1594 (-8.6824, -49.2404) -> (-10.822, -48.8148)
  line L1595 (-45.3154, 21.1309) -> (-44.3505, 23.0874)
  line L1596 (12.941, 48.2963) -> (15.0353, 47.6858)
  line L1597 (0, 50) -> (0, 0)
  line L1598 (-32.1394, 38.3022) -> (-30.4381, 39.6677)
  line L1599 (-15.0353, 47.6858) -> (-12.941, 48.2963)
  line L1600 (38.3022, 32.1394) -> (39.6677, 30.4381)
  line L1601 (-48.8148, 10.822) -> (-48.2963, 12.941)
  line L1602 (-46.194, 19.1342) -> (-45.3154, 21.1309)
  line L1603 (35.3553, 35.3553) -> (36.8639, 33.7795)
  line L1604 (23.0874, 44.3505) -> (25, 43.3013)
  line L1605 (-33.7795, -36.8639) -> (-35.3553, -35.3553)
  line L1606 (33.7795, 36.8639) -> (35.3553, 35.3553)
  line L1607 (-17.101, -46.9846) -> (-19.1342, -46.194)
  line L1608 (-19.1342, -46.194) -> (-21.1309, -45.3154)
  line L1609 (25, 43.3013) -> (26.865, 42.1696)
  line L1610 (-26.865, -42.1696) -> (-28.6788, -40.9576)
  line L1611 (-23.0874, -44.3505) -> (-25, -43.3013)
  line L1612 (-28.6788, -40.9576) -> (-30.4381, -39.6677)
  line L1613 (30.4381, 39.6677) -> (32.1394, 38.3022)
  line L1614 (32.1394, 38.3022) -> (33.7795, 36.8639)
  line L1615 (-25, -43.3013) -> (-26.865, -42.1696)
  line L1616 (4.3578, -49.8097) -> (2.181, -49.9524)
  line L1617 (0, 50) -> (2.181, 49.9524)
  line L1618 (2.181, 49.9524) -> (4.3578, 49.8097)
  line L1619 (2.181, -49.9524) -> (0, -50)
  line L1620 (4.3578, 49.8097) -> (6.5263, 49.5722)
  line L1621 (6.5263, -49.5722) -> (4.3578, -49.8097)
  line L1622 (0, 0) -> (0, 50)
  line L1623 (-36.8639, 33.7795) -> (-35.3553, 35.3553)
  line L1624 (-33.7795, 36.8639) -> (-32.1394, 38.3022)
  line L1625 (-40.9576, 28.6788) -> (-39.6677, 30.4381)
  line L1626 (-32.1394, 38.3022) -> (-30.4381, 39.6677)
  line L1627 (-28.6788, 40.9576) -> (-26.865, 42.1696)
  line L1628 (-26.865, 42.1696) -> (-25, 43.3013)
  line L1629 (-38.3022, 32.1394) -> (-36.8639, 33.7795)
  line L1630 (-45.3154, 21.1309) -> (-44.3505, 23.0874)
  line L1631 (-42.1696, 26.865) -> (-40.9576, 28.6788)
  line L1632 (-44.3505, 23.0874) -> (-43.3013, 25)
  line L1633 (-30.4381, 39.6677) -> (-28.6788, 40.9576)
  line L1634 (-46.194, 19.1342) -> (-45.3154, 21.1309)
  line L1635 (-35.3553, 35.3553) -> (-33.7795, 36.8639)
  line L1636 (-39.6677, 30.4381) -> (-38.3022, 32.1394)
  line L1637 (-46.9846, 17.101) -> (-46.194, 19.1342)
  line L1638 (-43.3013, 25) -> (-42.1696, 26.865)
  line L1639 (-25, 43.3013) -> (-23.0874, 44.3505)
  line L1640 (0, -50) -> (-2.181, -49.9524)
  line L1641 (-47.6858, 15.0353) -> (-46.9846, 17.101)
  line L1642 (-2.181, -49.9524) -> (-4.3578, -49.8097)
  line L1643 (-4.3578, -49.8097) -> (-6.5263, -49.5722)
  line L1644 (-36.8639, -33.7795) -> (-38.3022, -32.1394)
  line L1645 (-35.3553, -35.3553) -> (-36.8639, -33.7795)
  line L1646 (-32.1394, -38.3022) -> (-33.7795, -36.8639)
  line L1647 (-30.4381, -39.6677) -> (-32.1394, -38.3022)
  line L1648 (-33.7795, -36.8639) -> (-35.3553, -35.3553)
  line L1649 (-28.6788, -40.9576) -> (-30.4381, -39.6677)
  line L1650 (-23.0874, -44.3505) -> (-25, -43.3013)
  line L1651 (-21.1309, -45.3154) -> (-23.0874, -44.3505)
  line L1652 (-25, -43.3013) -> (-26.865, -42.1696)
  line L1653 (-8.6824, -49.2404) -> (-10.822, -48.8148)
  line L1654 (-10.822, -48.8148) -> (-12.941, -48.2963)
  line L1655 (-17.101, -46.9846) -> (-19.1342, -46.194)
  line L1656 (-26.865, -42.1696) -> (-28.6788, -40.9576)
  line L1657 (-12.941, -48.2963) -> (-15.0353, -47.6858)
  line L1658 (-15.0353, -47.6858) -> (-17.101, -46.9846)
  line L1659 (-19.1342, -46.194) -> (-21.1309, -45.3154)
  line L1660 (-6.5263, -49.5722) -> (-8.6824, -49.2404)
  line L1661 (23.0874, 44.3505) -> (25, 43.3013)
  line L1662 (25, 43.3013) -> (26.865, 42.1696)
  line L1663 (30.4381, 39.6677) -> (32.1394, 38.3022)
  line L1664 (26.865, 42.1696) -> (28.6788, 40.9576)
  line L1665 (28.6788, 40.9576) -> (30.4381, 39.6677)
  line L1666 (-23.0874, 44.3505) -> (-21.1309, 45.3154)
  line L1667 (-17.101, 46.9846) -> (-15.0353, 47.6858)
  line L1668 (-12.941, 48.2963) -> (-10.822, 48.8148)
  line L1669 (4.3578, 49.8097) -> (6.5263, 49.5722)
  line L1670 (-10.822, 48.8148) -> (-8.6824, 49.2404)
  line L1671 (12.941, 48.2963) -> (15.0353, 47.6858)
  line L1672 (-21.1309, 45.3154) -> (-19.1342, 46.194)
  line L1673 (0, 50) -> (2.181, 49.9524)
  line L1674 (8.6824, 49.2404) -> (10.822, 48.8148)
  line L1675 (-15.0353, 47.6858) -> (-12.941, 48.2963)
  line L1676 (6.5263, 49.5722) -> (8.6824, 49.2404)
  line L1677 (-4.3578, 49.8097) -> (-2.181, 49.9524)
  line L1678 (-8.6824, 49.2404) -> (-6.5263, 49.5722)
  line L1679 (10.822, 48.8148) -> (12.941, 48.2963)
  line L1680 (-19.1342, 46.194) -> (-17.101, 46.9846)
  line L1681 (-2.181, 49.9524) -> (0, 50)
  line L1682 (15.0353, 47.6858) -> (17.101, 46.9846)
  line L1683 (2.181, 49.9524) -> (4.3578, 49.8097)
  line L1684 (-6.5263, 49.5722) -> (-4.3578, 49.8097)
  line L1685 (17.101, 46.9846) -> (19.1342, 46.194)
  line L1686 (21.1309, 45.3154) -> (23.0874, 44.3505)
  line L1687 (19.1342, 46.194) -> (21.1309, 45.3154)
sketch "Sketch3" plane through (0, 0, 0) normal (0, 0, 1) x (1, 0, 0)
  line L0 (60, 60) -> (-60, 60)
  line L1 (-60, 60) -> (-60, -60)
  line L2 (-60, -60) -> (60, -60)
  line L3 (60, -60) -> (60, 60)
  line L4 (60, 60) -> (-60, -60) construction
  line L5 (-60, 60) -> (60, -60) construction
  dimension "d1" = 120
  dimension "d2" = 120
  constraint horizontal L0
  constraint perpendicular L0 L1
  constraint parallel L0 L2
  constraint parallel L1 L3
  constraint coincident L4 origin
  constraint coincident L5 origin
  measures "d1" distance of L0.start L0.end
  measures "d2" distance of L0.end L1.end
extrude "Extrude1" add sketch "Sketch3" along normal blind 10 makes body 1
sketch "Sketch4" plane through (0, 0, 10) normal (0, 0, 1) x (-1, 0, 0)
  line L0 (-60, 60) -> (-60, -60)
  line L1 (-60, -60) -> (60, -60)
  line L2 (60, -60) -> (60, 60)
  line L3 (60, 60) -> (-60, 60)
  circle A0 centre (0, 0) radius 50
  line L4 (60, -60) -> (55.889, -60)
  line L5 (48.2857, 60) -> (60, 60)
  line L6 (60, 60) -> (60, -60)
  line L7 (55.889, -60) -> (-60, -60)
  line L8 (-60, -60) -> (-60, -55)
  line L9 (-60, -55) -> (55.889, -55)
  line L10 (55.889, -55) -> (55.889, -60)
  line L11 (-60, -55) -> (-55, -55)
  line L12 (-55, -55) -> (-55, 60)
  line L13 (-55, 60) -> (-60, 60)
  line L14 (-60, 60) -> (-60, -55)
  circle A1 centre (0, 0) radius 55
  line L15 (-16.25, -47.2857) -> (16.25, -47.2857)
  line L16 (-26.3342, -48.2857) -> (26.3342, -48.2857)
  line L17 (60, 60) -> (55, 60)
  line L18 (55, 60) -> (55, -60)
  line L19 (55, -60) -> (60, -60)
  line L20 (60, -60) -> (60, 60)
  dimension "d7" = 55
  dimension "d8" = 55
  dimension "d9" = 110
  dimension "d34" = 32.5
  dimension "d35" = 1
  constraint coincident A0.centre A1.centre
  constraint horizontal L4
  constraint horizontal L5
  constraint vertical L6
  constraint coincident L3 L5.start
  constraint coincident L1.end L2.start
  constraint horizontal L7
  constraint vertical L8
  constraint horizontal L9
  constraint vertical L10
  constraint coincident L0 L8.end
  constraint horizontal L11
  constraint vertical L12
  constraint horizontal L13
  constraint vertical L14
  constraint coincident L3 L12.end
  constraint coincident A0 L15.start
  constraint coincident A0 L15.end
  constraint horizontal L15
  constraint coincident A1 L16.start
  constraint coincident A1 L16.end
  constraint parallel L15 L16
  constraint horizontal L17
  constraint vertical L18
  constraint horizontal L19
  constraint vertical L20
  constraint coincident L4 L18.end
  constraint coincident L2.end L3.start
  measures "d7" distance of A0.centre L12
  measures "d8" distance of A0.centre L9
  measures "d9" diameter of A1
  measures "d34" distance of L15.start L15.end
  measures "d35" distance of L15 L16
extrude "Extrude2" cut sketch "Sketch4" against normal blind 5 contours L3 L5 L12 A1 L18 | A0 A1 L16 | A0 L15 L16 | A0 L15 picked at (-53.0822, 3.9751) bodies 1
sketch "Sketch5" plane through (0, 0, 5) normal (0, 0, 1) x (-1, 0, 0)
  line L0 (55, 60) -> (-55, 60)
  line L1 (-55, 60) -> (-55, 0)
  line L2 (15, 60) -> (-15, 60)
  line L3 (-15, 60) -> (-15, 35)
  line L4 (-15, 35) -> (15, 35)
  line L5 (15, 35) -> (15, 60)
  arc A0 (-55, 0) -> (-26.3342, -48.2857) centre (0, 0) ccw
  line L6 (-26.3342, -48.2857) -> (26.3342, -48.2857)
  arc A1 (26.3342, -48.2857) -> (55, 0) centre (0, 0) ccw
  line L7 (55, 0) -> (55, 60)
  dimension "d12" = 30
  dimension "d13" = 15
  dimension "d14" = 25
  constraint horizontal L2
  constraint vertical L3
  constraint horizontal L4
  constraint vertical L5
  constraint coincident L0 L2.start
  measures "d12" distance of L3 L5
  measures "d13" distance of A0.centre L5
  measures "d14" distance of L2 L4
extrude "Extrude3" cut sketch "Sketch5" against normal blind 5 contours L0 L2 L3 L4 L5 bodies 1
sketch "Sketch6" plane through (0, 0, 5) normal (0, 0, 1) x (-1, 0, 0)
  line L0 (-15, 35) -> (-15, 60)
  line L1 (-15, 60) -> (-55, 60)
  line L2 (-55, 60) -> (-55, 0)
  line L3 (55, 60) -> (15, 60)
  line L4 (15, 60) -> (15, 35)
  line L5 (15, 35) -> (-15, 35)
  line L6 (-0.5, -60) -> (0.5, -60)
  line L7 (0.5, -60) -> (0.5, 60)
  line L8 (0.5, 60) -> (-0.5, 60)
  line L9 (-0.5, 60) -> (-0.5, -60)
  line L10 (-0.5, -60) -> (0.5, 60) construction
  line L11 (0.5, -60) -> (-0.5, 60) construction
  arc A0 (-55, 0) -> (-26.3342, -48.2857) centre (0, 0) ccw
  line L12 (-26.3342, -48.2857) -> (26.3342, -48.2857)
  arc A1 (26.3342, -48.2857) -> (55, 0) centre (0, 0) ccw
  line L13 (55, 0) -> (55, 60)
  dimension "d17" = 1
  dimension "d18" = 120
  constraint horizontal L6
  constraint perpendicular L6 L7
  constraint parallel L6 L8
  constraint parallel L7 L9
  constraint coincident L10 A0.centre
  constraint coincident L11 A0.centre
  measures "d17" distance of L7 L9
  measures "d18" distance of L6.start L8.end
extrude "Extrude4" add sketch "Sketch6" along normal blind 1 contours L5 L7 L9 L12 | L6 L7 L9 L12 bodies 1
chamfer "Chamfer1" distance 0.5 angle 45 2 edges at (0.5, 6.6429, 6) (-0.5, 6.6429, 6) on bodies 1
fillet "Fillet1" radius 60 1 edges at (60, 60, 5) on bodies 1
fillet "Fillet1" radius 60 1 edges at (-60, 60, 5) on bodies 1
fillet "Fillet2" radius 5 2 edges at (-15, -60, 2.5) (15, -60, 2.5) on bodies 1
copy_body "Body->Comp1" bodies 1 removing the originals makes body 2 in component "base"
sketch "Sketch1" plane through (0, 0, 5) normal (0, 0, 1) x (-1, 0, 0) in component "top"
  arc A0 (-15, 55) -> (-20, 60) centre (-20, 55) ccw
  line L0 (-20, 60) -> (-55, 60)
  line L1 (-55, 60) -> (-55, 0)
  line L2 (-0.5, -48.2857) -> (-0.5, 35)
  line L3 (-0.5, 35) -> (-15, 35)
  line L4 (-15, 35) -> (-15, 55)
  line L5 (-49, 3) -> (-30.9925, 3)
  line L6 (-30.9925, 3) -> (-30.9925, -3)
  line L7 (-30.9925, -3) -> (-49, -3)
  line L8 (-49, -3) -> (-49, 3)
  line L9 (-49, 16) -> (-43, 16)
  line L10 (-43, 16) -> (-43, -16)
  line L11 (-43, -16) -> (-49, -16)
  line L12 (-49, -16) -> (-49, 16)
  line L13 (-33, 28) -> (-31, 28)
  line L14 (-31, 28) -> (-31, -28)
  line L15 (-31, -28) -> (-33, -28)
  line L16 (-33, -28) -> (-33, 28)
  line L17 (49, -16) -> (43, -16)
  line L18 (30.9925, 3) -> (49, 3)
  line L19 (43, 16) -> (49, 16)
  line L20 (33, -28) -> (31, -28)
  line L21 (49, -3) -> (30.9925, -3)
  line L22 (30.9925, -3) -> (30.9925, 3)
  line L23 (49, 3) -> (49, -3)
  line L24 (31, -28) -> (31, 28)
  line L25 (33, 28) -> (33, -28)
  line L26 (49, 16) -> (49, -16)
  line L27 (43, -16) -> (43, 16)
  line L28 (31, 28) -> (33, 28)
  arc A1 (-55, 0) -> (-26.3342, -48.2857) centre (0, 0) ccw
  line L29 (-26.3342, -48.2857) -> (-0.5, -48.2857)
  constraint horizontal L5
  constraint vertical L6
  constraint horizontal L7
  constraint vertical L8
  constraint horizontal L9
  constraint vertical L10
  constraint horizontal L11
  constraint vertical L12
  constraint horizontal L13
  constraint vertical L14
  constraint horizontal L15
  constraint vertical L16
extrude "Extrude1'" add sketch "Sketch1" along normal blind 5 separate body contours L5 L9 L10 L12 | L5 L7 L8 L10 L12 | L5 L7 L10 L16 | L7 L10 L11 L12 | L5 L7 L14 L16 | L17 L21 L26 L27 | L18 L21 L23 L26 L27 | L18 L21 L25 L27 | L18 L19 L26 L27 | L18 L21 L24 L25 makes body 3 at (47, -1, 5) makes body 4 at (-47, -1, 5) in component "top"
sketch "Sketch2" plane through (0, 0, 10) normal (0, 0, 1) x (-1, 0, 0) in component "top"
  line L0 (-31, -3) -> (-31, 3)
  line L1 (-31, 3) -> (-43, 3)
  line L2 (-43, 3) -> (-43, 16)
  line L3 (-43, 16) -> (-49, 16)
  line L4 (-49, 16) -> (-49, -16)
  line L5 (-49, -16) -> (-43, -16)
  line L6 (-43, -16) -> (-43, -3)
  line L7 (-43, -3) -> (-31, -3)
  line L8 (-49, 3) -> (49, 3)
  line L9 (49, 3) -> (49, -3)
  line L10 (49, -3) -> (-49, -3)
  line L11 (-49, -3) -> (-49, 3)
  constraint horizontal L8
  constraint vertical L9
  constraint horizontal L10
  constraint vertical L11
  constraint coincident L4 L8.start
extrude "Extrude2'" add sketch "Sketch2" 1 faces at (-47, 1, 10) along normal blind 5 on bodies 4 bodies 3 4 in component "top"
sketch "Sketch3 (2)" plane through (0, 0, 15) normal (0, 0, 1) x (-1, 0, 0) in component "top"
  line L0 (43, 3) -> (-43, 3)
  line L1 (-43, 3) -> (-43, 16)
  line L2 (-43, 16) -> (-49, 16)
  line L3 (-49, 16) -> (-49, -16)
  line L4 (-49, -16) -> (-43, -16)
  line L5 (-43, -16) -> (-43, -3)
  line L6 (-43, -3) -> (43, -3)
  line L7 (43, -3) -> (43, -16)
  line L8 (43, -16) -> (49, -16)
  line L9 (49, -16) -> (49, 16)
  line L10 (49, 16) -> (43, 16)
  line L11 (43, 16) -> (43, 3)
  line L12 (-11, -3) -> (11, -3)
  line L13 (11, -3) -> (11, 3)
  line L14 (11, 3) -> (-11, 3)
  line L15 (-11, 3) -> (-11, -3)
  constraint horizontal L12
  constraint vertical L13
  constraint horizontal L14
  constraint vertical L15
  constraint coincident L0 L13.end
  constraint coincident L6 L12.start
extrude "Extrude3'" add sketch "Sketch3 (2)" along normal blind 20 contours L0 L6 L12 L13 L14 L15 bodies 3 in component "top"
fillet "Fillet1'" radius 4 2 edges at (-11, 0, 35) (11, 0, 35) on bodies 3 in component "top"
sketch "Sketch4 (2)" plane through (0, -3, 0) normal (0, -1, 0) x (1, 0, 0) in component "top"
  arc A0 (11, 31) -> (7, 35) centre (7, 31) ccw
  line L0 (7, 35) -> (-7, 35)
  arc A1 (-7, 35) -> (-11, 31) centre (-7, 31) ccw
  line L1 (-11, 31) -> (-11, 15)
  line L2 (-11, 15) -> (-43, 15)
  line L3 (-43, 15) -> (-43, 5)
  line L4 (-43, 5) -> (-31, 5)
  line L5 (-31, 5) -> (-31, 10)
  line L6 (-31, 10) -> (31, 10)
  line L7 (31, 10) -> (31, 5)
  line L8 (31, 5) -> (43, 5)
  line L9 (43, 5) -> (43, 15)
  line L10 (43, 15) -> (11, 15)
  line L11 (11, 15) -> (11, 31)